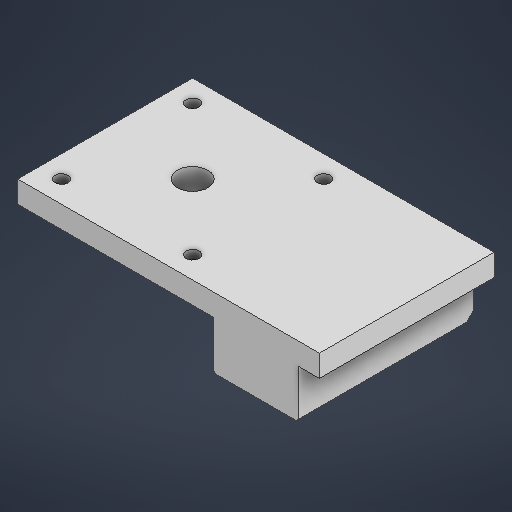
# Autodesk Inventor part: Tensioner Top
Saved by Autodesk Inventor 2025.1 (Build 291241000, 241)
## iProperties
Created: 2025-02-02
Part Number: Tensioner Top
Material: Generic
Document SubType Name: Modeling
Designer: jerem
Density: 1 g/cm^3
Appearance: Default
Author: jerem
## iProperties of the stored document Tensioner Top_3DPrint.ipt
Created: 2025-02-02
Part Number: Tensioner Top_3DPrint
Material: Generic
Document SubType Name: Modeling
Designer: jerem
Density: 1 g/cm^3
Appearance: Default
Author: jerem
Autodesk Inventor part; units mm, degrees
ref_plane "YZ Plane" through (0, 0, 0) normal (1, 0, 0) x (0, 1, 0)
ref_plane "XZ Plane" through (0, 0, 0) normal (0, 1, 0) x (-1, 0, 0)
ref_plane "XY Plane" through (0, 0, 0) normal (0, 0, 1) x (1, 0, 0)
sketch "Sketch1" plane through (0, 0, 0) normal (0, 1, 0) x (-1, 0, 0)
  line L0 (-20, 20) -> (20, 20)
  line L1 (20, 20) -> (20, -20)
  line L2 (20, -20) -> (-20, -20)
  line L3 (-20, -20) -> (-20, 20)
  line L4 (-20, 20) -> (20, -20) construction
  line L5 (20, 20) -> (-20, -20) construction
  circle A0 centre (15, -15) radius 1.5
  circle A1 centre (-15, -15) radius 1.5
  circle A2 centre (-15, 15) radius 1.5
  circle A3 centre (15, 15) radius 1.5
  line L6 (15, 15) -> (15, -15) construction
  line L7 (-15, -15) -> (15, -15) construction
  line L8 (-15, -15) -> (-15, 15) construction
  line L9 (-20, 20) -> (-49, 20)
  line L10 (-49, 20) -> (-49, -20)
  line L11 (-49, -20) -> (-20, -20)
  line L12 (-24.8, -20) -> (-24.8, 20)
  line L13 (-44.2, 20) -> (-44.2, -20)
  line L14 (-24.8, 15) -> (-44.2, 15)
  line L15 (-27.8, -20) -> (-27.8, 12)
  line L16 (-27.8, 12) -> (-41.2, 12)
  line L17 (-41.2, 12) -> (-41.2, -20)
  circle A4 centre (0, 0) radius 3.5
  line L18 (-24.8, 15) -> (-20, 15) construction
  line L19 (-44.2, 15) -> (-49, 15) construction
  dimension "d0" = 40
  dimension "d1" = 40
  dimension "d2" = 30
  dimension "d3" = 3
  dimension "d6" = 19.4
  dimension "d7" = 5
  dimension "d12" = 3
  dimension "d13" = 3
  dimension "d14" = 3
  dimension "d26" = 7
  dimension "d27" = 29
  constraints: 40 end point, 15 point on line, 11 perpendicular, 5 centre point, 3 equal radius, 3 parallel, 2 equal length, 2 horizontal, 2 midpoint, 1 coincident, 1 vertical
  measures "d0" distance of L1.end L2.end
  measures "d1" distance of L0.end L1.end
  measures "d2" distance of L7.start L6.end
  measures "d3" diameter of A0
  measures "d6" distance between parallel lines of L12 L13
  measures "d7" distance between parallel lines of L9 L14
  measures "d12" distance between parallel lines of L12 L15
  measures "d13" distance between parallel lines of L14 L16
  measures "d14" distance between parallel lines of L13 L17
  measures "d26" diameter of A4
  measures "d27" distance between parallel lines of L10 L3
extrude "Extrusion1" add sketch "Sketch1" along normal blind 5
extrude "Extrusion2" add sketch "Sketch1" against normal blind 11 contours L12 L14 L13 L9 | L11 L15 L16 L17 L13 L14 L12
extrude "Extrusion3" add sketch "Sketch1" against normal blind 3 contours L11 L17 L16 L15
chamfer "Chamfer1" distance 2 angle 45 3 edges at (27.8, -3, -4) (34.5, -3, 12) (41.2, -3, -4)
chamfer "Chamfer2" distance 2 angle 45 2 edges at (26.3, -11, -20) (42.7, -11, -20)
chamfer "Chamfer3" distance 0.5 angle 45 2 edges at (24.8, -11, 1) (44.2, -11, 1)
equation "\"d13\" = d12"
equation "\"d14\" = d12"
body "Solid1"
